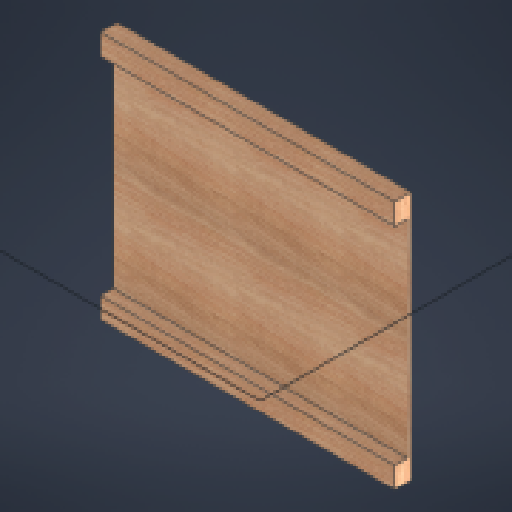
# Autodesk Inventor part: Drawer
Saved by Autodesk Inventor 2023.2 (Build 272271030, 271C)
## iProperties
Created: 2023-02-22
Part Number: Drawer
Material: Holz (Birke)
Document SubType Name: Modeling
Designer: Stefan
Mass: 3465 g
Surface Area: 9560 cm^2
Volume: 6300 cm^3
Density: 0.55 g/cm^3
Appearance: Birke - natur - poliert
Author: Stefan
Autodesk Inventor part; units mm, degrees
ref_plane "YZ Plane" through (0, 0, 0) normal (1, 0, 0) x (0, 1, 0)
ref_plane "XZ Plane" through (0, 0, 0) normal (0, 1, 0) x (-1, 0, 0)
ref_plane "XY Plane" through (0, 0, 0) normal (0, 0, 1) x (1, 0, 0)
sketch "Skizze1" plane through (0, 0, 0) normal (1, 0, 0) x (0, 1, 0)
  line L0 (300, 30) -> (250, 30)
  line L1 (250, 30) -> (250, 0)
  line L2 (250, 0) -> (300, 0)
  line L3 (300, 0) -> (300, 30)
  line L4 (-250, 30) -> (-300, 30)
  line L5 (-300, 30) -> (-300, 0)
  line L6 (-300, 0) -> (-250, 0)
  line L7 (-250, 0) -> (-250, 30)
  line L8 (300, 0) -> (-300, 0)
  line L9 (-300, 0) -> (-300, -10)
  line L10 (-300, -10) -> (300, -10)
  line L11 (300, -10) -> (300, 0)
  point P0 (0, 0)
  point P1 (0, 0)
  point P2 (250, 0)
  point P3 (-250, 0)
  dimension "d0" = 50
  dimension "d1" = 30
  dimension "d2" = 600
  dimension "d3" = 10
  constraints: 24 end point, 6 parallel, 3 horizontal, 3 perpendicular, 2 equal length, 2 point on line, 1 coincident, 1 midpoint
  measures "d0" distance of L0.start L0.end
  measures "d1" distance of L2.end L0.start
  measures "d2" distance of L9.end L10.end
  measures "d3" distance of L8.end L9.end
extrude "Extrusion1" add sketch "Skizze1" along normal mid plane 700
